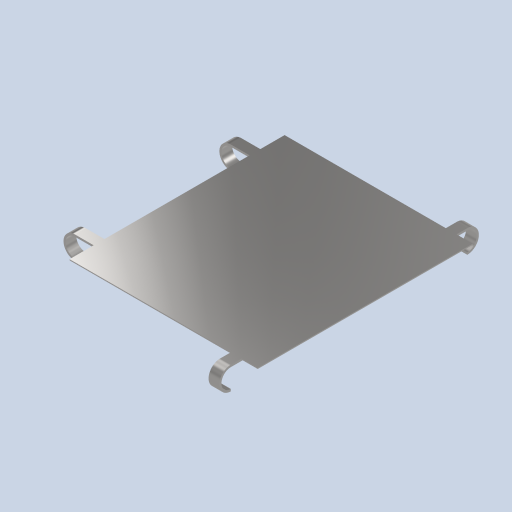
# Autodesk Inventor part: Part7
Saved by Autodesk Inventor 2024 (Build 280153000, 153)
## iProperties
Created: 2024-05-29
Part Number: Part7
Material: Generic
Document SubType Name: Modeling
Designer: mirun
Density: 1 g/cm^3
Appearance: Galvanized
Author: mirun
Autodesk Inventor part; units mm, degrees
ref_plane "YZ Plane" through (0, 0, 0) normal (1, 0, 0) x (0, 1, 0)
ref_plane "XZ Plane" through (0, 0, 0) normal (0, 1, 0) x (-1, 0, 0)
ref_plane "XY Plane" through (0, 0, 0) normal (0, 0, 1) x (1, 0, 0)
sketch "Sketch1" plane through (0, 0, 0) normal (0, 1, 0) x (-1, 0, 0)
  line L0 (-175, 200) -> (175, 200)
  line L1 (175, 200) -> (175, -200)
  line L2 (175, -200) -> (-175, -200)
  line L3 (-175, -200) -> (-175, 200)
  line L4 (-175, 200) -> (175, -200) construction
  line L5 (175, 200) -> (-175, -200) construction
  point P0 (0, 0)
  point P1 (0, 0)
  dimension "d0" = 350
  dimension "d1" = 400
  constraints: 12 end point, 2 midpoint, 2 parallel, 1 coincident, 1 horizontal, 1 perpendicular
  measures "d0" distance of L0.start L0.end
  measures "d1" distance of L0.end L1.end
extrude "Extrusion1" add sketch "Sketch1" along normal blind 2
sketch "Sketch2" plane through (0, 0, 0) normal (0, -1, 0) x (1, 0, 0)
  line L0 (175, 200) -> (175, -200) construction
  line L1 (-175, 200) -> (175, 200) construction
  line L2 (175, 155) -> (125, 155)
  line L3 (125, 155) -> (125, 135)
  line L4 (125, 135) -> (175, 135)
  line L5 (175, 135) -> (175, 155)
  line L6 (0, 0) -> (119.5058, 0) construction
  line L7 (175, -155) -> (125, -155)
  line L8 (125, -155) -> (125, -135)
  line L9 (125, -135) -> (175, -135)
  line L10 (175, -135) -> (175, -155)
  line L11 (175, -200) -> (-175, -200) construction
  line L12 (0, 0) -> (0, 102.1582) construction
  line L13 (-175, 155) -> (-125, 155)
  line L14 (-125, 155) -> (-125, 135)
  line L15 (-125, 135) -> (-175, 135)
  line L16 (-175, 135) -> (-175, 155)
  line L17 (-175, -155) -> (-125, -155)
  line L18 (-125, -155) -> (-125, -135)
  line L19 (-125, -135) -> (-175, -135)
  line L20 (-175, -135) -> (-175, -155)
  line L21 (125, 135) -> (145, 135)
  line L22 (145, 135) -> (145, 200)
  line L23 (145, 200) -> (125, 200)
  line L24 (125, 200) -> (125, 135)
  line L25 (125, -135) -> (145, -135)
  line L26 (145, -135) -> (145, -200)
  line L27 (145, -200) -> (125, -200)
  line L28 (125, -200) -> (125, -135)
  point P0 (150, 155)
  point P1 (150, -155)
  point P2 (-150, 155)
  point P3 (-150, -155)
  dimension "d4" = 50
  dimension "d5" = 20
  dimension "d6" = 45
  dimension "d9" = 20
  dimension "d10" = 20
  constraints: 52 end point, 15 symmetric about line, 6 parallel, 4 horizontal, 3 perpendicular, 3 point on line, 1 midpoint, 1 vertical
  measures "d4" distance of L4.end L3.end
  measures "d5" distance from line of point (150, 155) L4
  measures "d6" distance between parallel lines of L1 L2
  measures "d9" distance of L23.end L22.end
  measures "d10" distance of L26.end L27.end
extrude "Extrusion2" add sketch "Sketch2" along normal blind 2 contours L22 L4 L3 L2 | L2 L24 L23 L22 | L26 L27 L28 L7 | L7 L8 L9 L26 | L13 L14 L15 L16 | L20 L19 L18 L17
sketch "Sketch3" plane through (145, 0, 200) normal (1, 0, 0) x (0, 0, -1)
  line L0 (400, 2) -> (0, 2) construction
  line L1 (0, 2) -> (-20, 2)
  line L2 (0, -2) -> (-20, -2)
  line L3 (-20, -2) -> (-20, 2)
  arc A0 (-20, -2) -> (-20, -37) centre (-20, -19.5) ccw
  line L4 (-20, -2) -> (-20, -37) construction
  line L5 (-20, -2) -> (15, -2) construction
  arc A1 (-20, 2) -> (-20, -41) centre (-20, -19.5) ccw
  line L6 (-20, 2) -> (-20, -44.4597)
  line L7 (0, 2) -> (0, -2)
  point P0 (200, 0)
  point P1 (-20, -41)
  point P2 (-20, -37)
  dimension "d11" = 20
  dimension "d12" = 35
  dimension "d13" = 90
  dimension "d14" = 4
  constraints: 14 end point, 4 point on circle, 3 horizontal, 3 perpendicular, 2 centre point, 2 tangent, 1 point on line, 1 vertical
  measures "d11" distance of L0.end L1.end
  measures "d12" distance of L2.end L4.end
  measures "d13" angle of L4 L5
  measures "d14" distance of A1.end L4.end
extrude "Extrusion3" add sketch "Sketch3" against normal up to surface (20 mm away) contours L7 L2 L3 L1 | L3 A0 L6 A1
mirror "Mirror1" about plane through (0, 0, 0) normal (0, 0, 1) of "Extrusion3"
sketch "Sketch4" plane through (-175, 0, 155) normal (0, 0, 1) x (1, 0, 0)
  line L0 (139.9111, 57.1289) -> (-260.0889, 57.1289) construction
  line L1 (0, 1.8433) -> (-35, 1.8433)
  line L2 (0, -2) -> (-35, -2)
  line L3 (-35, -2) -> (-35, 1.8433)
  arc A0 (-35, -2) -> (-35, -37) centre (-35, -19.5) ccw
  line L4 (-35, -2) -> (-35, -37) construction
  line L5 (-280.0889, 53.1289) -> (-245.0889, 53.1289) construction
  arc A1 (-35, 1.8433) -> (-35, -41) centre (-35, -19.5784) ccw
  line L6 (-35, 1.8433) -> (-35, -44.4597)
  line L7 (0, 1.8433) -> (0, -2)
  point P0 (175, 0)
  point P1 (-60.0889, 55.1289)
  point P2 (-280.0889, 14.1289)
  point P3 (-280.0889, 18.1289)
  point P4 (-35, -37)
  point P5 (-35, -2)
  point P6 (-35, -2)
  dimension "d17" = 35
  dimension "d18" = 35
  dimension "d19" = 90
  dimension "d20" = 4
  constraints: 16 end point, 4 point on circle, 3 horizontal, 3 perpendicular, 2 centre point, 2 tangent, 1 point on line, 1 vertical
  measures "d17" distance of L1.start L1.end
  measures "d18" distance of L2.end L4.end
  measures "d19" angle of L4 L5
  measures "d20" distance of A1.end L4.end
extrude "Extrusion4" add sketch "Sketch4" against normal up to surface (20 mm away) contours L7 L2 L3 L1 | L3 A0 L6 A1
mirror "Mirror2" about plane through (0, 0, 0) normal (0, 0, 1) of "Extrusion4"
body "Solid1"
